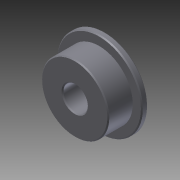
# Autodesk Inventor part: 0.25 in Flanged Ball Bearing
Saved by Autodesk Inventor 2014 SP1 (Build 180222100, 222)
## iProperties
Created: 2012-03-04
Part Number: 0.25 in Flanged Ball Bearing
Material: Steel
Document SubType Name: Modeling
Designer: Moses
Mass: 14.7404 g
Surface Area: 12.9515 cm^2
Volume: 1.87776 cm^3
Density: 7.85 g/cm^3
Appearance: Steel
Author: Moses
Autodesk Inventor part; units mm, degrees
ref_plane "YZ Plane" through (0, 0, 0) normal (1, 0, 0) x (0, 1, 0)
ref_plane "XZ Plane" through (0, 0, 0) normal (0, 1, 0) x (-1, 0, 0)
ref_plane "XY Plane" through (0, 0, 0) normal (0, 0, 1) x (1, 0, 0)
sketch "Sketch1" plane through (0, 0, 0) normal (0, 0, 1) x (1, 0, 0)
  circle A0 centre (0, 0) radius 8.7313
  circle A1 centre (0, 0) radius 11.1125
  circle A2 centre (0, 0) radius 3.175
  dimension "d0" = 17.4625
  dimension "d1" = 22.225
  dimension "d2" = 6.35
  constraints: 3 centre point, 3 coincident
  measures "d0" diameter of A0
  measures "d1" diameter of A1
  measures "d2" diameter of A2
extrude "Extrusion1" add sketch "Sketch1" along normal blind 6.35 contours A0
extrude "Extrusion2" add sketch "Sketch1" against normal blind 1.5875 contours A0 | A1
chamfer "Chamfer1" distance 0.254 angle 45 5 edges at (-8.7313, 0, 6.35) (-11.1125, 0, 0) (-11.1125, 0, -1.5875) (-3.175, 0, 6.35) (-3.175, 0, -1.5875)
body "Solid1"
